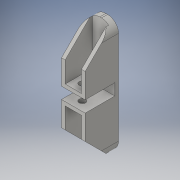
# Autodesk Inventor part: Control board Holder
Saved by Autodesk Inventor 2016 (Build 200138000, 138)
## iProperties
Created: 2017-10-10
Part Number: Control board Holder
Material: Generic
Document SubType Name: Modeling
Designer: Student
Density: 1 g/cm^3
Appearance: Default
Author: Student
Autodesk Inventor part; units mm, degrees
ref_plane "YZ Plane" through (0, 0, 0) normal (1, 0, 0) x (0, 1, 0)
ref_plane "XZ Plane" through (0, 0, 0) normal (0, 1, 0) x (-1, 0, 0)
ref_plane "XY Plane" through (0, 0, 0) normal (0, 0, 1) x (1, 0, 0)
sketch "Sketch1" plane through (0, 0, 0) normal (0, 0, 1) x (1, 0, 0)
  line L0 (-7.182, 9.0471) -> (3.8416, 9.0471)
  line L1 (3.8416, 9.0471) -> (3.8416, -44.5723)
  line L2 (3.8416, -44.5723) -> (-7.182, -44.5723)
  line L3 (-7.182, -44.5723) -> (-7.182, 9.0471)
  point P0 (0, 0)
  dimension "d0" = 11.0236
  dimension "d1" = 53.6194
  constraints: 8 end point, 2 parallel, 1 horizontal, 1 perpendicular
  measures "d0" distance of L0.start L0.end
  measures "d1" distance of L0.end L1.end
extrude "Extrusion1" add sketch "Sketch1" along normal blind 1.7018
sketch "Sketch2" plane through (0, 0, 1.7018) normal (0, 0, 1) x (1, 0, 0)
  line L0 (3.8416, 9.0471) -> (-7.182, 9.0471) projected
  line L1 (3.8416, -44.5723) -> (3.8416, 9.0471) projected
  line L2 (-7.182, 9.0471) -> (3.8416, 9.0471)
  line L3 (3.8416, 9.0471) -> (3.8416, -15.0829)
  line L4 (3.8416, -15.0829) -> (-7.182, -15.0829)
  line L5 (-7.182, -15.0829) -> (-7.182, 9.0471)
  point P0 (0, 0)
  dimension "d4" = 24.13
  constraints: 8 end point, 2 parallel, 1 horizontal, 1 perpendicular, 1 point on line
  measures "d4" distance of L4.end L0.end
extrude "Extrusion2" add sketch "Sketch2" along normal blind 13.843
sketch "Sketch3" plane through (-7.182, 9.0471, 0) normal (0, 1, 0) x (1, 0, 0)
  circle A0 centre (5.5118, -11.3348) radius 1.5
  line L0 (11.0236, -15.5448) -> (0, -15.5448) projected
  point P0 (7.182, 0)
  dimension "d7" = 3
  dimension "d8" = 4.21
  constraints: 1 centre point
  measures "d7" diameter of A0
  measures "d8" distance from line of A0.centre L0
extrude "Extrusion3" cut sketch "Sketch3" against normal blind 25.4
chamfer "Chamfer1" distance 12.7 angle 45 1 edges at (-1.6702, 9.0471, 15.5448)
sketch "Sketch4" plane through (-7.182, 9.0471, 0) normal (0, 1, 0) x (1, 0, 0)
  line L0 (11.0236, -2.8448) -> (0, -2.8448) projected
  line L1 (0, -15.5448) -> (11.0236, -15.5448) projected
  line L2 (1.7272, -2.8448) -> (9.2964, -2.8448)
  line L3 (9.2964, -2.8448) -> (9.2964, -15.5448)
  line L4 (9.2964, -15.5448) -> (1.7272, -15.5448)
  line L5 (1.7272, -15.5448) -> (1.7272, -2.8448)
  point P0 (7.182, 0)
  dimension "d14" = 1.7272
  dimension "d15" = 1.7272
  constraints: 8 end point, 3 point on line, 2 parallel, 1 horizontal, 1 perpendicular
  measures "d14" distance of L0.end L2.start
  measures "d15" distance of L0.start point (9.296, -2.845)
extrude "Extrusion4" cut sketch "Sketch4" against normal blind 22.4028
sketch "Sketch5" plane through (0, 0, 1.7018) normal (0, 0, 1) x (1, 0, 0)
  line L0 (-7.182, -44.5723) -> (3.8416, -44.5723) projected
  line L1 (3.8416, 9.0471) -> (3.8416, -44.5723) projected
  line L2 (-7.182, -44.5723) -> (3.8416, -44.5723)
  line L3 (3.8416, -44.5723) -> (3.8416, -20.4423)
  line L4 (3.8416, -20.4423) -> (-7.182, -20.4423)
  line L5 (-7.182, -20.4423) -> (-7.182, -44.5723)
  point P0 (0, 0)
  dimension "d18" = 24.13
  constraints: 8 end point, 2 parallel, 1 horizontal, 1 perpendicular, 1 point on line
  measures "d18" distance of L4.end L0.start
extrude "Extrusion5" add sketch "Sketch5" along normal blind 13.843
sketch "Sketch6" plane through (-7.182, -44.5723, 0) normal (0, -1, 0) x (1, 0, 0)
  circle A0 centre (5.5118, 11.3348) radius 1.5 projected
  circle A1 centre (5.5118, 11.3348) radius 1.5
  point P0 (7.182, 0)
  constraints: 1 centre point, 1 coincident
extrude "Extrusion6" cut sketch "Sketch6" against normal blind 39.243
chamfer "Chamfer2" distance 12.7 angle 45 1 edges at (-1.6702, -44.5723, 15.5448)
sketch "Sketch7" plane through (-7.182, -44.5723, 0) normal (0, -1, 0) x (1, 0, 0)
  line L0 (1.7272, 2.8448) -> (9.2964, 2.8448) projected
  line L1 (9.2964, 2.8448) -> (9.2964, 15.5448) projected
  line L2 (9.2964, 15.5448) -> (1.7272, 15.5448) projected
  line L3 (9.2964, 2.8448) -> (1.7272, 2.8448)
  line L4 (1.7272, 2.8448) -> (1.7272, 15.5448)
  line L5 (1.7272, 15.5448) -> (9.2964, 15.5448)
  line L6 (9.2964, 15.5448) -> (9.2964, 2.8448)
  point P0 (7.182, 0)
  constraints: 8 end point, 2 parallel, 1 coincident, 1 horizontal, 1 perpendicular
extrude "Extrusion7" cut sketch "Sketch7" against normal blind 22.4028
sketch "Sketch8" plane through (-5.4548, -44.5723, 2.8448) normal (0, 0, 1) x (1, 0, 0)
  circle A0 centre (3.7846, 11.2014) radius 1.5
  circle A1 centre (3.7846, 42.418) radius 1.5034
  line L0 (0, 0) -> (7.5692, 0) projected
  line L1 (7.5692, 53.6194) -> (0, 53.6194) projected
  point P0 (5.4548, 44.5723)
  dimension "d28" = 3
  dimension "d29" = 3.0067
  dimension "d30" = 11.2014
  dimension "d31" = 11.2014
  constraints: 2 centre point
  measures "d28" diameter of A0
  measures "d29" diameter of A1
  measures "d30" distance from line of A0.centre L0
  measures "d31" distance from line of A1.centre L1
extrude "Extrusion8" cut sketch "Sketch8" against normal blind 22.4028
fillet "Fillet1" radius 5.08 4 edges at (-7.182, 9.0471, 1.4224) (3.8416, 9.0471, 1.4224) (-7.182, -44.5723, 1.4224) (3.8416, -44.5723, 1.4224)
equation "\"d15\" = d14"
equation "\"d31\" = d30"
body "Solid1"
